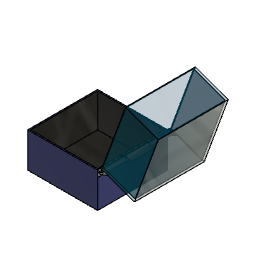
Hinged Box (Autodesk Fusion 360 design; units mm, degrees)
Autodesk Fusion 360 part; units mm, degrees
note: some values were not read from the file. Chosen so that the rebuilt part matches the saved one: which bodies a step acts on; which face or edge a step refers to. Set by a fixed rule: which sketch regions a step uses.
sketch "Box" plane through (0, 0, 0) normal (0, 0, 1) x (1, 0, 0) in component "Bottom Box"
  line L0 (0, 0) -> (-70, 0)
  line L1 (-70, 0) -> (-70, 70)
  line L2 (-70, 70) -> (0, 70)
  line L3 (0, 70) -> (0, 0)
  dimension "d1" = 70
  dimension "d2" = 70
  constraint horizontal L0
  constraint vertical L1
  constraint horizontal L2
  constraint vertical L3
  constraint coincident L0.start L3.end
  measures "d1" distance of L0.start L0.end
  measures "d2" distance of L0.start L2.end
extrude "Extrude1" add sketch "Box" along normal blind 70 makes body 1 in component "Bottom Box"
shell "Shell1" thickness 1.3 removed faces 0 bodies 1 in component "Bottom Box"
ref_plane "WorkPlane1" through (-35, 35, 35) normal (0, 0, 1) x (1, 0, 0) in component "Bottom Box"
split "Split1" by plane through (-35, 35, 35) normal (0, 0, 1) bodies 1 makes body 2 at (-23.3333, 23.3333, 70) in component "Bottom Box"
sketch "Hinge" plane through (0, 0, 0) normal (0, -1, 0) x (1, 0, 0) in component "Bottom Box"
  line L0 (0, 35) -> (-70, 35)
  line L1 (-70, 35) -> (-70, 0)
  line L2 (-70, 0) -> (0, 0)
  line L3 (0, 0) -> (0, 35)
  line L4 (0, 35) -> (2.95, 35)
  circle A0 centre (2.95, 35) radius 2.45
  circle A1 centre (2.95, 35) radius 1.15
  circle A2 centre (2.95, 35) radius 0.65
  line L5 (0, 28.5852) -> (4.6824, 33.2676)
  line L6 (0, 41.4148) -> (4.6824, 36.7324)
  line L7 (0, 35) -> (0, 41.4148)
  line L8 (0, 28.5852) -> (0, 35)
  dimension "d10" = 2.95
  dimension "d11" = 1.3
  dimension "d12" = 0.5
  dimension "d13" = 1.3
  dimension "d14" = 45
  dimension "d15" = 45
  constraint coincident L0.start L3.end
  constraint perpendicular L3 L4
  constraint coincident L4.end A0.centre
  constraint concentric A0 A1
  constraint concentric A1 A2
  constraint coincident L3 L5.start
  constraint coincident A0 L5.end
  constraint tangent A0 L5
  constraint coincident A0 L6.end
  constraint tangent A0 L6
  constraint perpendicular L0 L7
  measures "d10" distance of L0.start L4.end
  measures "d11" diameter of A2
  measures "d12" distance of A1 A2
  measures "d13" distance of A0 A1
  measures "d14" angle of L3 L5
  measures "d15" angle of L6 L7
extrude "Extrude2" add sketch "Hinge" against normal up to surface (70 mm away) separate body contours L3 L4 A0 L5 L8 | A0 makes body 3 in component "Bottom Box"
extrude "Extrude3" add sketch "Hinge" against normal up to surface (70 mm away) separate body contours L4 A0 L6 L7 | A0 | A1 | A2 makes body 4 in component "Bottom Box"
extrude "Extrude4" add sketch "Hinge" against normal up to surface (70 mm away) separate body contours A2 makes body 5 in component "Bottom Box"
sketch "Sketch3" plane through (0, 0, 35) normal (0, 0, 1) x (-1, 0, 0) in component "Bottom Box"
  line L0 (0, 0) -> (0, -70)
  line L1 (0, -70) -> (70, -70)
  line L2 (70, -70) -> (70, 0)
  line L3 (70, 0) -> (0, 0)
  line L4 (1.3, -68.7) -> (1.3, -1.3)
  line L5 (1.3, -1.3) -> (68.7, -1.3)
  line L6 (68.7, -1.3) -> (68.7, -68.7)
  line L7 (68.7, -68.7) -> (1.3, -68.7)
  line L8 (0, 0) -> (-5.5, 0)
  line L9 (-5.5, 0) -> (-5.5, -1.3)
  line L10 (-5.5, -1.3) -> (0, -1.3)
  line L11 (0, -1.3) -> (0, 0)
  line L12 (0, -1.3) -> (-5.5, -1.3)
  line L13 (-5.5, -1.3) -> (-5.5, -1.8)
  line L14 (-5.5, -1.8) -> (0, -1.8)
  line L15 (0, -1.8) -> (0, -1.3)
  line L16 (0, -35) -> (-10, -35) construction
  line L17 (0, -35) -> (0, -23.5) construction
  line L18 (0, -23.5) -> (-5.5, -23.5)
  line L19 (-5.5, -23.5) -> (-5.5, -23)
  line L20 (-5.5, -23) -> (0, -23)
  line L21 (0, -23) -> (0, -23.5)
  line L22 (-5.5, -46.5) -> (-5.5, -47)
  line L23 (-5.5, -70) -> (-5.5, -68.7)
  line L24 (-5.5, -68.7) -> (0, -68.7)
  line L25 (-5.5, -47) -> (0, -47)
  line L26 (0, -46.5) -> (-5.5, -46.5)
  line L27 (0, -68.7) -> (-5.5, -68.7)
  line L28 (0, -70) -> (-5.5, -70)
  line L29 (0, -68.7) -> (0, -70)
  line L30 (0, -68.2) -> (0, -68.7)
  line L31 (0, -47) -> (0, -46.5)
  line L32 (-5.5, -68.7) -> (-5.5, -68.2)
  line L33 (-5.5, -68.2) -> (0, -68.2)
  point P0 (0, -70)
  point P1 (0, -70)
  dimension "d22" = 5.5
  dimension "d23" = 1.3
  dimension "d24" = 0.5
  dimension "d25" = 11.5
  dimension "d26" = 5.5
  dimension "d27" = 0.5
  constraint horizontal L8
  constraint vertical L9
  constraint horizontal L10
  constraint vertical L11
  constraint coincident L0.start L3.end
  constraint horizontal L12
  constraint vertical L13
  constraint horizontal L14
  constraint vertical L15
  constraint coincident L9 L13.end
  constraint midpoint L0 L16.start
  constraint perpendicular L0 L16
  constraint coincident L0 L17.end
  constraint horizontal L18
  constraint vertical L19
  constraint horizontal L20
  constraint vertical L21
  constraint symmetric L0.start L16 P1
  constraint symmetric L0.start L16 P0
  constraint symmetric L8.end L16 L23.start
  constraint symmetric L9.end L16 L23.end
  constraint symmetric L10.end L16 L24.end
  constraint symmetric L13.end L16 L32.end
  constraint symmetric L14.end L16 L30.start
  constraint symmetric L16 L17.end L26.start
  constraint symmetric L16 L18.end L22.start
  constraint symmetric L16 L19.end L22.end
  constraint symmetric L16 L20.end L25.end
  measures "d22" distance of L0.start L8.end
  measures "d23" distance of L0.start L10.end
  measures "d24" distance of L10.end L14.end
  measures "d25" distance of L16.start L17.end
  measures "d26" distance of L17.end L18.end
  measures "d27" distance of L17.end L20.end
extrude "Extrude5" cut sketch "Sketch3" along normal through all and the other way through all contours L0 L10 L12 L13 L14 L15 | L0 L18 L19 L20 L21 | L0 L24 L27 L30 L32 L33 | L0 L22 L25 L26 L31 bodies 3 4 makes body 10 at (5.3585, 8.8667, 34.5512) makes body 11 at (1.7275, 1.3, 37.7157) makes body 12 at (5.3585, 31.1667, 34.5512) makes body 13 at (1.7275, 68.7, 37.7157) makes body 6 at (0.5029, 38.8333, 35.1187) makes body 7 at (0.5029, 15.9333, 35.1187) makes body 8 at (0.5029, 61.1333, 35.1187) makes body 9 at (0.7443, 0, 32.562) in component "Bottom Box"
delete_body "RemoveBody1" bodies 6 in component "Bottom Box"
delete_body "RemoveBody2" bodies 10 in component "Bottom Box"
delete_body "RemoveBody3" bodies 4 in component "Bottom Box"
copy_body "Body->Comp1" bodies 2 removing the originals makes body 14 in component "Top Box"
copy_body "CutPasteBodies1" bodies 5 11 12 13 removing the originals makes body 15 makes body 16 makes body 17 makes body 18 in component "Top Box"
component "Bottom Box" placed x (1, 0, 0) y (0, 1, 0) z (0, 0, 1) at (0, 0, 0)
component "Top Box" placed x (1, 0, 0) y (0, 1, 0) z (0, 0, 1) at (0, 0, 0)
equation "WallThickness = 1.3 mm" comment "FDM 3D Printer Thickness"
equation "BoxHeight = 70 mm"
equation "Gap = 0.5 mm"
equation "d6 = BoxHeight"
equation "d8 = WallThickness"
equation "d9 = -BoxHeight / 2"
equation "d11 = WallThickness"
equation "d12 = Gap"
equation "d13 = WallThickness"
equation "d23 = WallThickness"
equation "d24 = Gap"
equation "d27 = Gap"
named bodies: "Bottom Body", "Top Body", "Bottom Hinge", "Top Hinge", "Pin", "Bottom Hinge (1)", "Bottom Hinge (2)", "Bottom Hinge (3)", "Bottom Hinge (4)", "Top Hinge (1)", "Top Hinge (2)", "Top Hinge (3)", "Top Hinge (4)"
